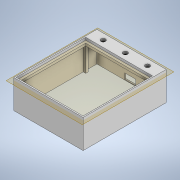
# Autodesk Inventor part: Mainbody2
Saved by Autodesk Inventor 2021 (Build 250183000, 183)
## iProperties
Created: 2021-05-04
Part Number: Mainbody2
Material: Generic
Document SubType Name: Modeling
Designer: email
Density: 1 g/cm^3
Appearance: Default
Author: email
Autodesk Inventor part; units mm, degrees
ref_plane "YZ Plane" through (0, 0, 0) normal (1, 0, 0) x (0, 1, 0)
ref_plane "XY Plane" through (0, 0, 0) normal (0, 0, 1) x (1, 0, 0)
sketch "Sketch1" plane through (0, 0, 0) normal (0, 1, 0) x (-1, 0, 0)
  line L0 (24.775, -25.7234) -> (-24.775, -25.7234)
  line L1 (-24.775, -25.7234) -> (-24.775, 25.7234)
  line L2 (-24.775, 25.7234) -> (24.775, 25.7234)
  line L3 (24.775, 25.7234) -> (24.775, -25.7234)
  line L4 (24.775, -25.7234) -> (-24.775, 25.7234) construction
  line L5 (-24.775, -25.7234) -> (24.775, 25.7234) construction
  line L6 (26.775, -27.8) -> (-26.775, -27.8)
  line L7 (-26.775, -27.8) -> (-26.775, 27.8)
  line L8 (-26.775, 27.8) -> (26.775, 27.8)
  line L9 (26.775, 27.8) -> (26.775, -27.8)
  line L10 (26.775, -27.8) -> (-26.775, 27.8) construction
  line L11 (-26.775, -27.8) -> (26.775, 27.8) construction
  line L12 (-26.775, -17.5745) -> (-24.775, -17.5745)
  line L13 (27.775, -28.8383) -> (-27.775, -28.8383)
  line L14 (-27.775, -28.8383) -> (-27.775, 28.8383)
  line L15 (-27.775, 28.8383) -> (27.775, 28.8383)
  line L16 (27.775, 28.8383) -> (27.775, -28.8383)
  line L17 (27.775, -28.8383) -> (-27.775, 28.8383) construction
  line L18 (-27.775, -28.8383) -> (27.775, 28.8383) construction
  line L19 (-27.775, -9.8151) -> (-26.775, -9.8151)
  line L20 (-7.9068, 27.8) -> (-7.9068, 28.8383)
  line L21 (27.775, -27.8) -> (27.775, -37.8)
  line L22 (27.775, -37.8) -> (-27.775, -37.8)
  line L23 (-27.775, -37.8) -> (-27.775, -27.8)
  line L24 (27.775, -37.8) -> (27.775, -32.8)
  line L25 (27.775, -32.8) -> (-27.775, -32.8)
  line L26 (27.775, -32.8) -> (15.7648, -32.8)
  line L27 (27.775, -32.8) -> (17.75, -32.8)
  circle A0 centre (17.75, -32.8) radius 1.825
  line L28 (-27.775, -32.8) -> (-17.75, -32.8)
  circle A1 centre (-17.75, -32.8) radius 1.825
  circle A2 centre (0, -32.8) radius 1.825
  point P0 (0, 0)
  point P1 (22.7625, -32.8)
  point P2 (21.7699, -32.8)
  point P3 (-22.7625, -32.8)
  point P4 (-27.775, -28.8383)
  dimension "d0" = 53.55
  dimension "d1" = 55.6
  dimension "d2" = 2
  dimension "d3" = 1
  dimension "d4" = 10
  dimension "d6" = 55.55
  dimension "d8" = 10.025
  dimension "d9" = 3.65
  dimension "d11" = 10.025
  dimension "d12" = 3.65
  dimension "d13" = 3.65
  constraints: 58 end point, 14 midpoint, 14 point on line, 6 horizontal, 6 parallel, 5 perpendicular, 3 centre point, 2 coincident, 1 collinear, 1 horizontal alignment, 1 vertical
  measures "d0" distance of L7.end L8.end
  measures "d1" distance of L6.end L7.end
  measures "d2" distance of L12.start L12.end
  measures "d3" distance of L19.start L19.end
  measures "d4" distance of L21.start L21.end
  measures "d6" distance of L21.end L22.end
  measures "d8" distance of L27.start L27.end
  measures "d9" diameter of A0
  measures "d11" distance of L28.start L28.end
  measures "d12" diameter of A1
  measures "d13" diameter of A2
extrude "Extrusion1" add sketch "Sketch1" against normal blind 25 contours L7 L6 L9 L8 L20 L15 L16 L13 L14 L19 | L19 L14 L15 L20 L8 L7 | L13 L21 L25 A0 A2 A1 L23 | L25 A1 A2 A0 L21 L22 L23
sketch "Sketch2" plane through (0, -25, 0) normal (0, -1, 0) x (1, 0, 0)
  line L0 (-26.775, -27.8) -> (-26.775, -36.8)
  line L1 (26.775, -27.8) -> (-26.775, -27.8) projected
  line L2 (-26.775, -36.8) -> (26.775, -36.8)
  line L3 (26.775, -36.8) -> (26.775, -27.8)
  line L4 (26.775, -27.8) -> (-26.775, -27.8)
  line L5 (-26.775, -27.8) -> (-26.775, -36.8)
  point P0 (0, 0)
  dimension "d16" = 9
  constraints: 10 end point, 2 parallel, 1 horizontal, 1 perpendicular, 1 vertical
  measures "d16" distance of L0.start L0.end
extrude "Extrusion2" cut sketch "Sketch2" against normal blind 23
ref_plane "Work Plane1" through (0, -2, 0) normal (0, 1, 0) x (-1, 0, 0)
sketch "Sketch3" plane through (0, -2, 0) normal (0, 1, 0) x (-1, 0, 0)
  line L0 (26.775, -27.8) -> (-26.775, -27.8) projected
  line L1 (-26.775, -27.8) -> (-26.775, 27.8) projected
  line L2 (26.775, -27.8) -> (-26.775, -27.8)
  line L3 (-26.775, -27.8) -> (-26.775, 27.8)
  line L4 (-26.775, 27.8) -> (26.775, 27.8)
  line L5 (26.775, 27.8) -> (26.775, -27.8)
  line L6 (24.75, 25.8) -> (-24.75, 25.8)
  line L7 (-24.75, 25.8) -> (-24.75, -25.8)
  line L8 (-24.75, -25.8) -> (24.75, -25.8)
  line L9 (24.75, -25.8) -> (24.75, 25.8)
  line L10 (24.75, 25.8) -> (-24.75, -25.8) construction
  line L11 (-24.75, 25.8) -> (24.75, -25.8) construction
  point P0 (0, 0)
  dimension "d20" = 49.5
  dimension "d21" = 51.6
  constraints: 20 end point, 4 parallel, 2 horizontal, 2 midpoint, 2 perpendicular
  measures "d20" distance of L7.end L8.end
  measures "d21" distance of L6.end L7.end
extrude "Extrusion3" add sketch "Sketch3" against normal blind 2
sketch "Sketch4" plane through (0, -4, 0) normal (0, -1, 0) x (1, 0, 0)
  line L0 (24.75, -25.8) -> (24.75, 25.8) projected
  line L1 (-26.775, -27.8) -> (26.775, -27.8) projected
  line L2 (24.75, -25.8) -> (26.775, -25.8)
  line L3 (26.775, -25.8) -> (26.775, -27.8)
  line L4 (26.775, -27.8) -> (24.75, -27.8)
  line L5 (24.75, -27.8) -> (24.75, -25.8)
  line L6 (24.75, 25.8) -> (-24.75, 25.8) projected
  line L7 (-26.775, 27.8) -> (26.775, 27.8) projected
  line L8 (24.75, 25.8) -> (26.775, 25.8)
  line L9 (26.775, 25.8) -> (26.775, 27.8)
  line L10 (26.775, 27.8) -> (24.75, 27.8)
  line L11 (24.75, 27.8) -> (24.75, 25.8)
  line L12 (-24.75, 25.8) -> (-26.775, 25.8)
  line L13 (-26.775, 25.8) -> (-26.775, 27.8)
  line L14 (-26.775, 27.8) -> (-24.75, 27.8)
  line L15 (-24.75, 27.8) -> (-24.75, 25.8)
  line L16 (-24.75, -25.8) -> (-24.75, 25.8) projected
  line L17 (-24.75, -25.8) -> (-26.775, -25.8)
  line L18 (-26.775, -25.8) -> (-26.775, -27.8)
  line L19 (-26.775, -27.8) -> (-24.75, -27.8)
  line L20 (-24.75, -27.8) -> (-24.75, -25.8)
  point P0 (0, 0)
  constraints: 32 end point, 8 parallel, 4 horizontal, 4 perpendicular
extrude "Extrusion4" add sketch "Sketch4" along normal blind 21 contours L2 L3 L1 L5 | L11 L7 L9 L8 | L12 L13 L7 L15 | L1 L18 L17 L20
sketch "Sketch5" plane through (27.775, 0, -37.8) normal (0, 0, -1) x (-1, 0, 0)
  line L0 (52.525, -25) -> (3.025, -25) projected
  line L1 (0, 0) -> (55.55, 0) projected
  line L2 (27.775, -18) -> (32.275, -18)
  line L3 (27.775, -18) -> (23.275, -18)
  line L4 (23.275, -18) -> (23.275, -22.5)
  line L5 (32.275, -18) -> (32.275, -22.5)
  line L6 (23.275, -22.5) -> (32.275, -22.5)
  point P0 (27.775, 0)
  point P1 (27.775, 0)
  dimension "d29" = 4.5
  dimension "d30" = 4.5
  dimension "d34" = 4.5
  dimension "d35" = 4.5
  constraints: 10 end point, 2 horizontal, 2 vertical, 1 midpoint
  measures "d29" distance of L2.start L2.end
  measures "d30" distance of L2.start L3.end
  measures "d34" distance of L3.end L4.end
  measures "d35" distance of L2.end L5.end
sketch "Sketch6" plane through (0, -25, 0) normal (0, -1, 0) x (1, 0, 0)
  line L0 (-27.775, -37.8) -> (27.775, -37.8) projected
  line L1 (27.775, -37.8) -> (27.775, 28.8383) projected
  line L2 (-27.775, -37.8) -> (27.775, -37.8)
  line L3 (27.775, -37.8) -> (27.775, 28.8383)
  line L4 (27.775, 28.8383) -> (-27.775, 28.8383)
  line L5 (-27.775, 28.8383) -> (-27.775, -37.8)
  point P0 (0, 0)
  constraints: 8 end point, 2 parallel, 1 horizontal, 1 perpendicular
extrude "Extrusion5" cut sketch "Sketch6" against normal blind 2
extrude "Extrusion6" cut sketch "Sketch5" against normal blind 2
body "Solid1"
